Bielle sup 2 (Autodesk Fusion 360 design; units mm, degrees)
Autodesk Fusion 360 part; units mm, degrees
sketch "Sketch1" plane through (0, 0, 0) normal (0, 0, 1) x (1, 0, 0)
  line L0 (8.65, -8.65) -> (-8.65, -8.65)
  line L1 (-8.65, -8.65) -> (-8.65, 8.65)
  line L2 (-8.65, 8.65) -> (8.65, 8.65)
  line L3 (8.65, 8.65) -> (8.65, -8.65)
  line L4 (8.65, -8.65) -> (-8.65, 8.65) construction
  line L5 (-8.65, -8.65) -> (8.65, 8.65) construction
  circle A0 centre (0, 0) radius 3.25
  line L6 (-8.65, 8.65) -> (8.65, 8.65)
  line L7 (8.65, 8.65) -> (8.65, 6.65)
  line L8 (8.65, 6.65) -> (-8.65, 6.65)
  line L9 (-8.65, 6.65) -> (-8.65, 8.65)
  line L10 (-8.65, -8.65) -> (8.65, -8.65)
  line L11 (8.65, -8.65) -> (8.65, -6.65)
  line L12 (8.65, -6.65) -> (-8.65, -6.65)
  line L13 (-8.65, -6.65) -> (-8.65, -8.65)
  dimension "d4" = 6.5
  dimension "d10" = 2
  dimension "d11" = 2
  dimension "d12" = 13.3
  constraint horizontal L0
  constraint perpendicular L0 L1
  constraint parallel L0 L2
  constraint parallel L1 L3
  constraint coincident L4 A0.centre
  constraint coincident L5 A0.centre
  constraint coincident A0.centre origin
  constraint horizontal L6
  constraint vertical L7
  constraint horizontal L8
  constraint vertical L9
  constraint coincident L3 L7.end
  constraint horizontal L10
  constraint vertical L11
  constraint horizontal L12
  constraint vertical L13
  constraint coincident L3 L11.end
  measures "d4" diameter of A0
  measures "d10" distance of L6 L8
  measures "d11" distance of L0 L12
  measures "d12" distance of L8 L12
extrude "Extrude2" add sketch "Sketch1" against normal blind 12
extrude "Extrude3" add sketch "Sketch1" along normal blind 25 contours L0 L1 L3 L10 L11 L12 L13 | L1 L2 L3 L6 L7 L8 L9
fillet "Fillet1" radius 8.5 4 edges at (8.65, -7.65, 25) (-8.65, -7.65, 25) (-8.65, 7.65, 25) (8.65, 7.65, 25)
sketch "Sketch3" plane through (0, -8.65, 0) normal (0, -1, 0) x (1, 0, 0)
  arc A0 (-0.15, 25) -> (-8.65, 16.5) centre (-0.15, 16.5) ccw
  line L0 (-8.65, 16.5) -> (-8.65, -12)
  line L1 (-8.65, -12) -> (8.65, -12)
  line L2 (8.65, -12) -> (8.65, 16.5)
  arc A1 (8.65, 16.5) -> (0.15, 25) centre (0.15, 16.5) ccw
  line L3 (0.15, 25) -> (-0.15, 25)
  line L4 (-8.65, 16.5) -> (8.65, 16.5) construction
  line L5 (0, 0) -> (0, 16.5) construction
  circle A2 centre (0, 16.5) radius 2.1
  line L6 (8.65, 0) -> (-8.65, 0)
  dimension "d19" = 4.2
  dimension "d21" = 11.5
  constraint coincident A0.end L0.start
  constraint coincident L2.end A1.start
  constraint coincident L5.start origin
  constraint coincident L4 L5.end
  constraint perpendicular L4 L5
  constraint coincident L5.end A2.centre
  measures "d19" diameter of A2
extrude "Extrude4" cut sketch "Sketch3" against normal through all contours A2
sketch "Sketch7" plane through (8.65, 0, 0) normal (1, 0, 0) x (0, 1, 0)
  line L0 (8.65, 16.5) -> (6.65, 16.5)
  line L1 (6.65, 16.5) -> (6.65, 0)
  line L2 (6.65, 0) -> (-6.65, 0)
  line L3 (-6.65, 0) -> (-6.65, 16.5)
  line L4 (-6.65, 16.5) -> (-8.65, 16.5)
  line L5 (-8.65, 16.5) -> (-8.65, -12)
  line L6 (-8.65, -12) -> (8.65, -12)
  line L7 (8.65, -12) -> (8.65, 16.5)
  line L8 (0, 0) -> (8.65, 0) construction
  line L9 (8.65, 0) -> (-8.65, -12) construction
  line L10 (5.5, -9) -> (-5.5, -9)
  line L11 (-5.5, -9) -> (-5.5, -3)
  line L12 (-5.5, -3) -> (5.5, -3)
  line L13 (5.5, -3) -> (5.5, -9)
  line L14 (5.5, -9) -> (-5.5, -3) construction
  line L15 (-5.5, -9) -> (5.5, -3) construction
  point P0 (0, -6)
  dimension "d27" = 11
  dimension "d28" = 6
  constraint coincident L8.start origin
  constraint coincident L7 L8.end
  constraint perpendicular L7 L8
  constraint coincident L5.end L6.start
  constraint horizontal L10
  constraint perpendicular L10 L11
  constraint parallel L10 L12
  constraint parallel L11 L13
  constraint coincident L14 P0
  constraint coincident L15 P0
  constraint midpoint L9 P0
  measures "d27" distance of L11.end L12.end
  measures "d28" distance of L10.end L11.end
extrude "Extrude5" cut sketch "Sketch7" against normal blind 15 contours L10 L11 L12 L13
fillet "Fillet2" radius 6 2 edges at (0, 6.65, 0) (0, -6.65, 0)
named bodies: "Bielle sup 2"
